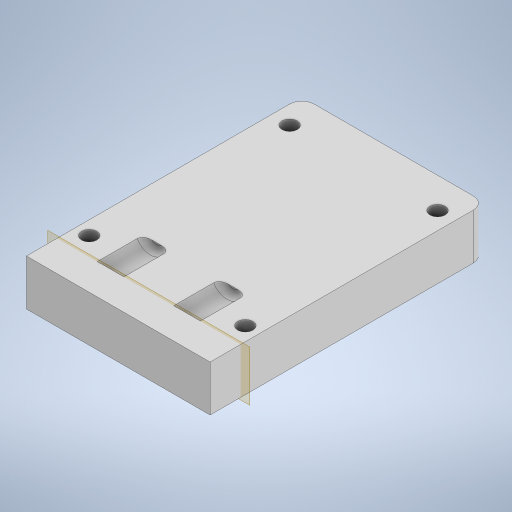
# Autodesk Inventor part: Adaptador_soporte_motor-rueda_error_asumido
Saved by Autodesk Inventor 2024 (Build 280153000, 153)
## iProperties
Created: 2023-03-15
Part Number: Adaptador_soporte_motor-rueda_error_asumido
Material: Generic
Document SubType Name: Modeling
Designer: Francisco
Density: 1 g/cm^3
Appearance: Default
Author: Francisco
Autodesk Inventor part; units mm, degrees
ref_plane "YZ Plane" through (0, 0, 0) normal (1, 0, 0) x (0, 1, 0)
ref_plane "XZ Plane" through (0, 0, 0) normal (0, 1, 0) x (-1, 0, 0)
ref_plane "XY Plane" through (0, 0, 0) normal (0, 0, 1) x (1, 0, 0)
sketch "Sketch1" plane through (0, 0, 0) normal (0, 1, 0) x (-1, 0, 0)
  line L0 (30, 45) -> (-30, 45)
  line L1 (-30, 45) -> (-30, -45)
  line L2 (-30, -45) -> (30, -45)
  line L3 (30, -45) -> (30, 45)
  line L4 (30, 45) -> (-30, -45) construction
  line L5 (-30, 45) -> (30, -45) construction
  point P0 (0, 0)
  dimension "d0" = 60
  dimension "d1" = 90
  constraints: 12 end point, 2 midpoint, 2 parallel, 1 horizontal, 1 perpendicular
  measures "d0" distance of L2.end L1.end
  measures "d1" distance of L1.end L0.end
extrude "Extrusion1" add sketch "Sketch1" along normal blind 15
sketch "Sketch2" plane through (0, 15, 0) normal (0, 1, 0) x (1, 0, 0)
  line L0 (-30, 45) -> (-30, -45) projected
  line L1 (-30, 45) -> (-20, 45)
  line L2 (-20, 45) -> (-20, 39)
  line L3 (-20, 39) -> (-30, 39)
  line L4 (-30, 39) -> (-30, 45)
  line L5 (30, -45) -> (30, 45) projected
  line L6 (30, 45) -> (20, 45)
  line L7 (20, 45) -> (20, 39)
  line L8 (20, 39) -> (30, 39)
  line L9 (30, 39) -> (30, 45)
  line L10 (30, -45) -> (25.5, -45)
  line L11 (25.5, -45) -> (25.5, -29)
  line L12 (25.5, -29) -> (30, -29)
  line L13 (30, -29) -> (30, -45)
  line L14 (-30, -45) -> (-25, -45)
  line L15 (-25, -45) -> (-25, -29)
  line L16 (-25, -29) -> (-30, -29)
  line L17 (-30, -29) -> (-30, -45)
  line L18 (30, 45) -> (-30, 45) projected
  line L19 (-30, 45) -> (-24, 45)
  line L20 (-24, 45) -> (-24, 35)
  line L21 (-24, 35) -> (-30, 35)
  line L22 (-30, 35) -> (-30, 45)
  line L23 (30, 45) -> (24.316, 45)
  line L24 (24.316, 45) -> (24.316, 35)
  line L25 (24.316, 35) -> (30, 35)
  line L26 (30, 35) -> (30, 45)
  line L27 (-30, -45) -> (30, -45) projected
  line L28 (-30, -45) -> (-25.5, -45)
  line L29 (-25.5, -45) -> (-25.5, -29)
  line L30 (-25.5, -29) -> (-30, -29)
  line L31 (-30, -29) -> (-30, -45)
  point P0 (0, 0)
  dimension "d4" = 10
  dimension "d5" = 6
  dimension "d6" = 10
  dimension "d7" = 4.5
  dimension "d8" = 16
  dimension "d17" = 6
  dimension "d18" = 10
  dimension "d19" = 5.684
  dimension "d20" = 10
  dimension "d21" = 4.5
  constraints: 56 end point, 14 parallel, 7 horizontal, 7 perpendicular, 3 point on line
  measures "d4" distance of L2.end L3.end
  measures "d5" distance of L1.end L2.end
  measures "d6" distance of L8.end L7.end
  measures "d7" distance of L11.end L12.end
  measures "d8" distance of L10.end L11.end
  measures "d17" distance of L20.end L21.end
  measures "d18" distance of L19.end L20.end
  measures "d19" distance of L25.end L24.end
  measures "d20" distance of L24.end L23.end
  measures "d21" distance of L30.end L29.end
fillet "Fillet1" radius 4 2 edges at (30, 7.5, -45) (-30, 7.5, -45)
hole "Hole2" at (-24, 15, -35) at (24.316, 15, -35) at (25.5, 15, 29) at (-25.5, 15, 29) direction (0, -1, 0) diameter 5 end through all
ref_plane "Work Plane2" through (-30, 0, 35) normal (0, 0, 1) x (1, 0, 0)
sketch "Sketch3" plane through (-30, 0, 35) normal (0, 0, 1) x (1, 0, 0)
  line L0 (0, 15) -> (17.5, 15)
  line L1 (2, 15) -> (7, 15) projected
  line L2 (17.5, 15) -> (17.5, 17.5)
  line L3 (17.5, 17.5) -> (42.5, 17.5)
  circle A0 centre (42.5, 17.5) radius 5
  circle A1 centre (17.5, 17.5) radius 5
  point P0 (30, 0)
  dimension "d31" = 17.5
  dimension "d32" = 2.5
  dimension "d33" = 25
  dimension "d34" = 10
  dimension "d35" = 10
  constraints: 6 end point, 2 centre point, 2 coincident, 1 collinear, 1 perpendicular, 1 vertical
  measures "d31" distance of L0.start L0.end
  measures "d32" distance of L0.end L2.end
  measures "d33" distance of L2.end L3.end
  measures "d34" diameter of A0
  measures "d35" diameter of A1
extrude "Extrusion2" cut sketch "Sketch3" against normal blind 15
fillet "Fillet2" radius 2 2 edges at (-12.5, 12.5, 20) (12.5, 12.5, 20)
body "Solid1"
